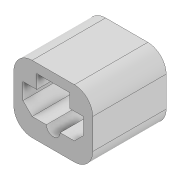
# Autodesk Inventor part: Cable_tie_connector_p1_metal
Saved by Autodesk Inventor 2022 (Build 260153000, 153)
## iProperties
Created: 2022-08-02
Part Number: Cable_tie_connector_p1_metal
Material: Generic
Document SubType Name: Modeling
Designer: dell
Density: 1 g/cm^3
Appearance: Default
Author: dell
Autodesk Inventor part; units mm, degrees
ref_plane "YZ Plane" through (0, 0, 0) normal (1, 0, 0) x (0, 1, 0)
ref_plane "XZ Plane" through (0, 0, 0) normal (0, 1, 0) x (-1, 0, 0)
ref_plane "XY Plane" through (0, 0, 0) normal (0, 0, 1) x (1, 0, 0)
sketch "Sketch1" plane through (0, 0, 0) normal (0, 0, 1) x (1, 0, 0)
  line L0 (-2.425, -0.3) -> (2.425, -0.3)
  line L1 (2.425, -0.3) -> (2.425, 0.3)
  line L2 (2.425, 0.3) -> (-2.425, 0.3)
  line L3 (-2.425, 0.3) -> (-2.425, -0.3)
  line L4 (-2.425, -0.3) -> (2.425, 0.3) construction
  line L5 (2.425, -0.3) -> (-2.425, 0.3) construction
  line L6 (-3.3, -2) -> (3.3, -2)
  line L7 (3.3, -2) -> (3.3, 2)
  line L8 (3.3, 2) -> (-3.3, 2)
  line L9 (-3.3, 2) -> (-3.3, -2)
  line L10 (-3.3, -2) -> (3.3, 2) construction
  line L11 (3.3, -2) -> (-3.3, 2) construction
  line L12 (-3.3, 0) -> (3.3, 0)
  line L13 (3.3, 0) -> (3.3, 2.3)
  line L14 (3.3, 2.3) -> (-3.3, 2.3)
  line L15 (-3.3, 2.3) -> (-3.3, 0)
  line L16 (-4.3, 3.3) -> (4.3, 3.3)
  line L17 (4.3, 3.3) -> (4.3, -4)
  line L18 (4.3, -4) -> (-4.3, -4)
  line L19 (-4.3, -4) -> (-4.3, 3.3)
  point P0 (0, 0)
  point P1 (-3.3, 2)
  point P2 (3.3, 2)
  dimension "d0" = 0.6
  dimension "d1" = 4.85
  dimension "d4" = 6.6
  dimension "d6" = 2
  dimension "d9" = 1
  dimension "d10" = 1
  dimension "d11" = 1
  dimension "d12" = 2
  dimension "d20" = 2
  constraints: 40 end point, 8 parallel, 6 midpoint, 4 perpendicular, 3 horizontal
  measures "d0" distance between parallel lines of L0 L2
  measures "d1" distance between parallel lines of L3 L1
  measures "d4" distance between parallel lines of L9 L7
  measures "d6" distance from line of point (0, 0) L6
  measures "d9" distance between parallel lines of L13 L17
  measures "d10" distance between parallel lines of L19 L15
  measures "d11" distance between parallel lines of L16 L14
  measures "d12" distance between parallel lines of L18 L6
  measures "d20" distance between parallel lines of L2 L14
extrude "Extrusion1" add sketch "Sketch1" along normal blind 3 contours L0 L1 L12 L7 L6 L9 L3 | L12 L9 L8 L7 L1 L2 L3 | L15 L14 L13 L8 | L16 L17 L18 L19
extrude "Extrusion2" add sketch "Sketch1" along normal blind 8
sketch "Sketch2" plane through (3.3, -2, 3) normal (-1, 0, 0) x (0, 0, 1)
  line L0 (0, 0) -> (0, 4.3) projected
  line L1 (0, 0) -> (5, 0) projected
  line L2 (5, 4.3) -> (5, 0) projected
  line L3 (0, 4.3) -> (5, 4.3) projected
  line L4 (0, 0) -> (0, 4.3) projected
  line L5 (0, 2.8) -> (4.1212, 4.3)
  line L6 (0, 4.3) -> (5, 4.3) projected
  point P0 (-3, 2)
  point P1 (0, 2.3)
  dimension "d22" = 0.5
  dimension "d23" = 70
  constraints: 2 end point, 2 point on line
  measures "d22" distance of point (0, 2.3) L5.start
  measures "d23" angle of L0 L5
extrude "Extrusion3" add sketch "Sketch2" along normal blind 7 contours L0 L3 L5
sketch "Sketch3" plane through (0, 0, 8) normal (0, 0, 1) x (1, 0, 0)
  line L0 (-4.3, -4) -> (4.3, -4) projected
  line L1 (4.3, -4) -> (4.3, 3.3) projected
  line L2 (4.3, 3.3) -> (-4.3, 3.3) projected
  line L3 (-4.3, 3.3) -> (-4.3, -4) projected
  line L4 (3.3, -2) -> (-3.3, -2) projected
  line L5 (-3.3, -2) -> (-3.3, 2.3) projected
  line L6 (-3.3, 2.3) -> (3.3, 2.3) projected
  line L7 (3.3, 2.3) -> (3.3, -2) projected
  line L8 (-3.3, 2.3) -> (-1.8, 2.3)
  line L9 (-1.8, 2.3) -> (-1.8, 0.8)
  line L10 (-1.8, 0.8) -> (-3.3, 0.8)
  line L11 (-3.3, 0.8) -> (-3.3, 2.3)
  line L12 (3.3, 2.3) -> (1.8, 2.3)
  line L13 (1.8, 2.3) -> (1.8, 0.8)
  line L14 (1.8, 0.8) -> (3.3, 0.8)
  line L15 (3.3, 0.8) -> (3.3, 2.3)
  point P0 (0, 0)
  point P1 (-3.3, 0.8)
  point P2 (-1.8, 2.3)
  dimension "d26" = 1.5
  dimension "d27" = 1.5
  dimension "d28" = 1.5
  dimension "d29" = 1.5
  constraints: 16 end point, 4 parallel, 2 horizontal, 2 perpendicular
  measures "d26" distance of L9.end L10.end
  measures "d27" distance of L8.end L9.end
  measures "d28" distance of L14.end L13.end
  measures "d29" distance of L13.end L12.end
extrude "Extrusion4" add sketch "Sketch3" against normal blind 5 contours L14 L13 L6 L7 | L5 L6 L9 L10
chamfer "Chamfer2" distance 1 angle 45 1 edges at (-3.3, -2, 5.5)
chamfer "Chamfer3" distance 1 angle 45 1 edges at (3.3, -2, 5.5)
sketch "Sketch4" plane through (0, 0, 8) normal (0, 0, 1) x (1, 0, 0)
  line L0 (-2.3, -2) -> (2.3, -2) projected
  circle A0 centre (0, -2) radius 0.75
  point P0 (0, 0)
  dimension "d39" = 1.5
  constraints: 1 centre point, 1 midpoint
  measures "d39" diameter of A0
extrude "Extrusion5" cut sketch "Sketch4" against normal blind 10
fillet "Fillet2" radius 2 4 edges at (-4.3, 3.3, 4) (4.3, 3.3, 4) (4.3, -4, 4) (-4.3, -4, 4)
body "Solid1"
